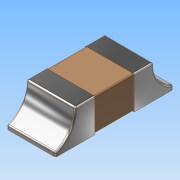
# Autodesk Inventor part: CL21A226MQCLQNC Capacitor
Saved by Autodesk Inventor 2016 (Build 200138000, 138)
## iProperties
Created: 2019-08-18
Part Number: CL21A226MQCLQNC Capacitor
Material: Laminate, Ivory, Matte
Document SubType Name: Modeling
Designer: Orest
Mass: 0.0033575 g
Surface Area: 0.126695 cm^2
Volume: 0.00243297 cm^3
Density: 1.38 g/cm^3
Appearance: Smooth - Ivory(1)
Author: Orest
Autodesk Inventor part; units mm, degrees
ref_plane "YZ Plane" through (0, 0, 0) normal (1, 0, 0) x (0, 1, 0)
ref_plane "XZ Plane" through (0, 0, 0) normal (0, 1, 0) x (-1, 0, 0)
ref_plane "XY Plane" through (0, 0, 0) normal (0, 0, 1) x (1, 0, 0)
sketch "Sketch10" plane through (0, 0, 0) normal (0, 0, 1) x (1, 0, 0)
  line L0 (-0.5, 0.4125) -> (0.5, 0.4125)
  line L1 (0.5, 0.4125) -> (0.5, -0.4125)
  line L2 (0.5, -0.4125) -> (-0.5, -0.4125)
  line L3 (-0.5, -0.4125) -> (-0.5, 0.4125)
  point P0 (0, 0)
  point P1 (-0.5, 0)
  point P2 (0, 0.4125)
  dimension "d7" = 1
  dimension "d8" = 0.825
  constraints: 8 end point, 2 midpoint, 2 parallel, 1 horizontal, 1 horizontal alignment, 1 perpendicular, 1 vertical alignment
  measures "d7" distance of L1.end L2.end
  measures "d8" distance of L0.end L1.end
extrude "Extrusion4" add sketch "Sketch10" along normal mid plane 1.225
sketch "Sketch11" plane through (0.5, -0.4125, 0.6125) normal (1, 0, 0) x (0, 0, -1)
  line L0 (0, 0.825) -> (1.225, 0.825) construction
  line L1 (0, 0) -> (0, 0.825) construction
  line L2 (0, 0) -> (1.225, 0) construction
  line L3 (1.225, 0.825) -> (1.225, 0) construction
  line L4 (1.2375, 0.8375) -> (-0.0125, 0.8375)
  line L5 (-0.0125, 0.8375) -> (-0.0125, -0.0125)
  line L6 (-0.0125, -0.0125) -> (1.2375, -0.0125)
  line L7 (1.2375, -0.0125) -> (1.2375, 0.8375)
  line L8 (-0.0125, -0.0125) -> (1.2375, -0.0125)
  line L9 (1.2375, -0.0125) -> (1.2375, 0.0875)
  line L10 (1.2375, 0.0875) -> (-0.0125, 0.0875)
  line L11 (-0.0125, 0.0875) -> (-0.0125, -0.0125)
  point P0 (0.6125, 0.4125)
  dimension "d11" = 1.25
  dimension "d14" = 0.1
  constraints: 16 end point, 2 parallel, 1 horizontal, 1 perpendicular, 1 point on line, 3 other
  measures "d11" distance of L4.start L4.end
  measures "d14" distance between parallel lines of L6 L10
extrude "Extrusion5" add sketch "Sketch11" along normal blind 0.5
extrude "Extrusion6" add sketch "Sketch11" along normal blind 1 contours L7 L6 L5 L10
fillet "Fillet1" radius 0.75 1 edges at (1, -0.325, 0)
fillet "Fillet2" radius 0.0425 10 edges at (0.75, 0.425, -0.625) (0.75, 0.425, 0.625) (1, 0.4036, 0.625) (1.1376, -0.0509, 0.625) (1, 0.4036, -0.625) (1.1376, -0.0509, -0.625) (1.5, -0.375, -0.625) (1.5, -0.325, 0) (1, 0.425, 0) (1.5, -0.375, 0.625)
mirror "Mirror1" about plane through (0, 0, 0) normal (1, 0, 0) of "Extrusion5", "Fillet1", "Fillet2", "Extrusion6"
fillet "Fillet3" radius 0.03 4 edges at (0, 0.4125, -0.6125) (0, 0.4125, 0.6125) (0, -0.4125, -0.6125) (0, -0.4125, 0.6125)
body "Solid4"
